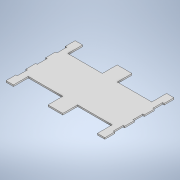
# Autodesk Inventor part: onderkant
Saved by Autodesk Inventor 2022 (Build 260153000, 153)
## iProperties
Created: 2022-01-28
Part Number: onderkant
Material: Generic
Document SubType Name: Modeling
Designer: keemi
Density: 1 g/cm^3
Appearance: Default
Author: keemi
Autodesk Inventor part; units mm, degrees
ref_plane "YZ Plane" through (0, 0, 0) normal (1, 0, 0) x (0, 1, 0)
ref_plane "XZ Plane" through (0, 0, 0) normal (0, 1, 0) x (-1, 0, 0)
ref_plane "XY Plane" through (0, 0, 0) normal (0, 0, 1) x (1, 0, 0)
sketch "Sketch1" plane through (0, 0, 0) normal (0, 1, 0) x (-1, 0, 0)
  line L0 (200, 0) -> (185, 0)
  line L1 (200, 0) -> (215, 0) construction
  line L2 (185, 0) -> (185, -30)
  line L3 (185, -30) -> (115, -30)
  line L4 (115, -30) -> (115, 0)
  line L5 (200, -140) -> (185, -140)
  line L6 (200, -140) -> (215, -140) construction
  line L7 (185, -140) -> (185, -110)
  line L8 (185, -110) -> (115, -110)
  line L9 (115, -110) -> (115, -140)
  line L10 (200, 0) -> (197, 0)
  line L11 (197, 0) -> (197, -140)
  line L12 (197, 0) -> (337, 0) construction
  line L13 (200, 0) -> (200, -20)
  line L14 (200, -20) -> (200, -40)
  line L15 (200, -40) -> (200, -60)
  line L16 (200, -60) -> (200, -80)
  line L17 (200, -80) -> (200, -100)
  line L18 (200, -100) -> (200, -120)
  line L19 (200, -120) -> (200, -140)
  line L20 (200, -20) -> (197, -20)
  line L21 (200, -40) -> (197, -40)
  line L22 (200, -60) -> (197, -60)
  line L23 (200, -80) -> (197, -80)
  line L24 (200, -100) -> (197, -100)
  line L25 (200, -120) -> (197, -120)
  line L26 (100, 0) -> (100, -140)
  line L27 (100, -140) -> (200, -140)
  line L28 (100, 0) -> (200, 0)
  line L29 (0, 0) -> (15, 0)
  line L30 (0, 0) -> (-15, 0) construction
  line L31 (15, 0) -> (15, -30)
  line L32 (15, -30) -> (85, -30)
  line L33 (85, -30) -> (85, 0)
  line L34 (85, -110) -> (85, -140)
  line L35 (15, -140) -> (15, -110)
  line L36 (15, -110) -> (85, -110)
  line L37 (0, -140) -> (15, -140)
  line L38 (0, -140) -> (-15, -140) construction
  line L39 (0, 0) -> (3, 0)
  line L40 (3, 0) -> (3, -140)
  line L41 (3, 0) -> (-137, 0) construction
  line L42 (0, 0) -> (0, -20)
  line L43 (0, -20) -> (0, -40)
  line L44 (0, -40) -> (0, -60)
  line L45 (0, -60) -> (0, -80)
  line L46 (0, -80) -> (0, -100)
  line L47 (0, -100) -> (0, -120)
  line L48 (0, -120) -> (0, -140)
  line L49 (0, -20) -> (3, -20)
  line L50 (0, -40) -> (3, -40)
  line L51 (0, -60) -> (3, -60)
  line L52 (0, -80) -> (3, -80)
  line L53 (0, -100) -> (3, -100)
  line L54 (0, -120) -> (3, -120)
  line L55 (100, -140) -> (0, -140)
  line L56 (100, 0) -> (0, 0)
  dimension "d2" = 15
  dimension "d3" = 180
  dimension "d4" = 30
  dimension "d5" = 70
  dimension "d6" = 90
  dimension "d12" = 3
  dimension "d13" = 140
  dimension "d14" = 90
  dimension "d15" = 20
  dimension "d16" = 20
  dimension "d17" = 20
  dimension "d18" = 20
  dimension "d19" = 20
  dimension "d20" = 20
  dimension "d21" = 20
  constraints: 114 end point, 27 symmetric about line, 22 point on line, 8 perpendicular, 3 horizontal, 2 collinear, 2 equal length, 2 vertical, 1 parallel
  measures "d2" distance of L0.start L0.end
  measures "d3" angle of L0 L1
  measures "d4" distance of L0.end L2.end
  measures "d5" distance of L2.end L3.end
  measures "d6" angle of L2 L3
  measures "d12" distance of L0.start L10.end
  measures "d13" distance of L10.end L11.end
  measures "d14" angle of L11 L12
  measures "d15" distance of L0.start L13.end
  measures "d16" distance of L13.end L14.end
  measures "d17" distance of L14.end L15.end
  measures "d18" distance of L15.end L16.end
  measures "d19" distance of L16.end L17.end
  measures "d20" distance of L17.end L18.end
  measures "d21" distance of L18.end L5.start
extrude "Extrusion1" add sketch "Sketch1" along normal blind 3 contours L13 L20 L11 L0 | L11 L5 L7 L8 L9 L27 L26 L28 L4 L3 L2 L0 | L15 L22 L11 L21 | L26 L55 L34 L36 L35 L37 L40 L29 L31 L32 L33 L56 | L17 L24 L11 L23 | L19 L5 L11 L25 | L40 L49 L42 L29 | L37 L48 L54 L40 | L40 L51 L44 L50 | L53 L46 L52 L40
body "Solid1"
